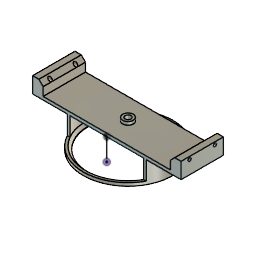
diancitiev4 (Autodesk Fusion 360 design; units mm, degrees)
part number: 2025-10-19-22-14-40-317
Autodesk Fusion 360 part; units mm, degrees
note: some values were not read from the file. Set by a fixed rule: which sketch regions a step uses.
sketch "Sketch1" plane through (0, 0, 0) normal (0, 0, 1) x (1, 0, 0)
  circle A0 centre (0, 0) radius 37.5
  circle A1 centre (0, 0) radius 42.25
  dimension "d1" = 75
  dimension "d26" = 84.5
  constraint coincident A0.centre A1.centre
  measures "d1" diameter of A0
  measures "d26" diameter of A1
extrude "Extrude1" add sketch "Sketch1" along normal blind 3
sketch "Sketch2" plane through (0, 0, 3) normal (0, 0, 1) x (-1, 0, 0)
  circle A0 centre (0, 0) radius 37.5
  circle A1 centre (0, 0) radius 42.25
  line L0 (-48.5856, 20) -> (48.5856, 20)
  line L1 (48.5856, 20) -> (48.5856, -20)
  line L2 (48.5856, -20) -> (-48.5856, -20)
  line L3 (-48.5856, -20) -> (-48.5856, 20)
  line L4 (-48.5856, 20) -> (48.5856, -20) construction
  line L5 (48.5856, 20) -> (-48.5856, -20) construction
  circle A2 centre (0, 0) radius 40
  circle A3 centre (0, 0) radius 43
  dimension "d4" = 40
  constraint horizontal L0
  constraint perpendicular L0 L1
  constraint parallel L0 L2
  constraint parallel L1 L3
  constraint coincident L4 A0.centre
  constraint coincident L5 A0.centre
  constraint coincident A0.centre A1.centre
  measures "d4" distance of L0.end L1.end
extrude "Extrude2" add sketch "Sketch2" along normal blind 17.5 contours A1 L0 L2 A2 | A1 L0 L2 A2
sketch "Sketch3" plane through (0, 0, 20.5) normal (0, 0, 1) x (-1, 0, 0)
  arc A0 (-37.2164, 20) -> (-37.2164, -20) centre (0, 0) ccw
  arc A1 (-34.641, 20) -> (-34.641, -20) centre (0, 0) ccw
  line L0 (-70, 20) -> (70, 20)
  line L1 (70, 20) -> (70, -20)
  line L2 (70, -20) -> (-70, -20)
  line L3 (-70, -20) -> (-70, 20)
  line L4 (-70, 20) -> (70, -20) construction
  line L5 (70, 20) -> (-70, -20) construction
  circle A2 centre (0, 0) radius 2.75
  line L6 (-34.641, 20) -> (-37.2164, 20)
  line L7 (-37.2164, -20) -> (-34.641, -20)
  dimension "d7" = 140
  dimension "d8" = 5.5
  dimension "d9" = 40
  constraint horizontal L0
  constraint perpendicular L0 L1
  constraint parallel L0 L2
  constraint parallel L1 L3
  constraint coincident L4 A0.centre
  constraint coincident L5 A0.centre
  constraint coincident A0.centre A1.centre
  constraint concentric A0 A2
  measures "d7" distance of L1.end L2.end
  measures "d8" diameter of A2
  measures "d9" distance of L0.start L2.end
extrude "Extrude3" add sketch "Sketch3" along normal blind 3
sketch "Sketch4" plane through (0, 0, 20.5) normal (0, 0, -1) x (1, 0, 0)
  arc A0 (-37.2164, 20) -> (-37.2164, -20) centre (0, 0) ccw
  line L0 (-37.2164, 20) -> (-70, 20)
  line L1 (-70, 20) -> (-70, -20)
  line L2 (-70, -20) -> (-37.2164, -20)
  line L3 (-70, 20) -> (-60, 20)
  line L4 (-60, 20) -> (-60, -20)
  line L5 (-60, -20) -> (-70, -20)
  line L6 (-70, -20) -> (-70, 20)
  line L7 (70, 20) -> (60, 20)
  line L8 (60, 20) -> (60, -20)
  line L9 (60, -20) -> (70, -20)
  line L10 (70, -20) -> (70, 20)
  dimension "d12" = 10
  constraint horizontal L3
  constraint vertical L4
  constraint horizontal L5
  constraint vertical L6
  constraint coincident L0.end L1.start
  constraint horizontal L7
  constraint vertical L8
  constraint horizontal L9
  constraint vertical L10
  measures "d12" distance of L0.end L3.end
extrude "Extrude4" add sketch "Sketch4" against normal blind 15 contours L0 L1 L2 L3 L4 L5 L6 | L7 L8 L9 L10
sketch "Sketch8" plane through (-70, 0, 0) normal (-1, 0, 0) x (0, -1, 0)
  line L0 (-20, 20.5) -> (20, 20.5)
  line L1 (20, 20.5) -> (20, 35.5)
  line L2 (20, 35.5) -> (-20, 35.5)
  line L3 (-20, 35.5) -> (-20, 20.5)
  line L4 (0, 0) -> (0, 33)
  line L5 (0, 33) -> (12, 33)
  line L6 (0, 33) -> (-12, 33)
  circle A0 centre (-12, 33) radius 1.5
  circle A1 centre (12, 33) radius 1.5
  circle A2 centre (-12, 33) radius 2.5
  circle A3 centre (12, 33) radius 2.5
  dimension "d31" = 33
  dimension "d32" = 12
  dimension "d33" = 12
  dimension "d34" = 3
  dimension "d35" = 3
  dimension "d36" = 5
  dimension "d37" = 5
  constraint coincident L4.start origin
  constraint perpendicular L0 L4
  constraint perpendicular L4 L5
  constraint perpendicular L4 L6
  constraint coincident L6.end A0.centre
  constraint coincident L5.end A1.centre
  constraint concentric A0 A2
  constraint concentric A1 A3
  measures "d31" distance of L4.start L4.end
  measures "d32" distance of L4.end L5.end
  measures "d33" distance of L4.end L6.end
  measures "d34" diameter of A0
  measures "d35" diameter of A1
  measures "d36" diameter of A2
  measures "d37" diameter of A3
extrude "Extrude7" cut sketch "Sketch8" against normal blind 151 contours A0 | A1
chamfer "Chamfer2" distance 4 angle 45 1 edges at (-60, 0, 35.5)
chamfer "Chamfer3" distance 4 angle 45 1 edges at (60, 0, 35.5)
sketch "Sketch9" plane through (70, 0, 0) normal (1, 0, 0) x (0, 1, 0)
  circle A0 centre (12, 33) radius 1.5
  circle A1 centre (-12, 33) radius 1.5
  line L0 (-20, 20.5) -> (20, 20.5)
  line L1 (20, 20.5) -> (20, 35.5)
  line L2 (20, 35.5) -> (-20, 35.5)
  line L3 (-20, 35.5) -> (-20, 20.5)
chamfer "Chamfer4" distance 2.5 angle 45 1 edges at (-34.9623, 13.5606, 3)
sketch "Sketch10" plane through (0, -20, 0) normal (0, -1, 0) x (1, 0, 0)
  line L0 (64, 35.5) -> (60, 31.5)
  line L1 (60, 31.5) -> (60, 23.5)
  line L2 (60, 23.5) -> (-60, 23.5)
  line L3 (-60, 23.5) -> (-60, 31.5)
  line L4 (-60, 31.5) -> (-64, 35.5)
  line L5 (-64, 35.5) -> (-70, 35.5)
  line L6 (-70, 35.5) -> (-70, 20.5)
  line L7 (-70, 20.5) -> (-37.2164, 20.5)
  line L8 (-37.2164, 20.5) -> (-37.2164, 3)
  line L9 (-37.2164, 3) -> (-34.641, 3)
  line L10 (-34.641, 3) -> (-34.641, 20.5)
  line L11 (-34.641, 20.5) -> (34.641, 20.5)
  line L12 (34.641, 20.5) -> (34.641, 3)
  line L13 (34.641, 3) -> (37.2164, 3)
  line L14 (37.2164, 3) -> (37.2164, 20.5)
  line L15 (37.2164, 20.5) -> (70, 20.5)
  line L16 (70, 20.5) -> (70, 35.5)
  line L17 (70, 35.5) -> (64, 35.5)
  line L18 (0, 0) -> (0, 20.5)
  dimension "d43" = 20.5
  constraint coincident L18.start origin
  constraint vertical L18
  measures "d43" distance of L18.start L18.end
sketch "Sketch11" plane through (0, 0, 20.5) normal (0, 0, -1) x (1, 0, 0)
  circle A0 centre (0, 0) radius 2.75
  arc A1 (-34.641, 20) -> (-34.641, -20) centre (0, 0) ccw
  line L0 (-34.641, -20) -> (34.641, -20)
  arc A2 (34.641, -20) -> (34.641, 20) centre (0, 0) ccw
  line L1 (34.641, 20) -> (-34.641, 20)
sketch "Sketch12" plane through (0, 0, 23.5) normal (0, 0, 1) x (-1, 0, 0)
  line L0 (60, -20) -> (60, 20)
  line L1 (60, 20) -> (-60, 20)
  line L2 (-60, 20) -> (-60, -20)
  line L3 (-60, -20) -> (60, -20)
  circle A0 centre (0, 0) radius 2.75
  circle A1 centre (0, 0) radius 2.75
  circle A2 centre (0, 0) radius 5
  dimension "d44" = 10
  constraint concentric A0 A1
  constraint concentric A0 A2
  measures "d44" diameter of A2
extrude "Extrude8" add sketch "Sketch12" along normal blind 3 contours A2
sketch "Sketch13" plane through (0, -20, 0) normal (0, -1, 0) x (1, 0, 0)
